rod_label_clip (Autodesk Fusion 360 design; units mm, degrees)
part number: 2026-09-05-07-00-16-324
Autodesk Fusion 360 part; units mm, degrees
sketch "Ring" plane through (0, 0, 0) normal (0, 1, 0) x (1, 0, 0)
  circle A0 centre (0, 0) radius 17.05
  circle A1 centre (0, 0) radius 19.45
extrude "Ring (1)" add sketch "Ring" along normal mid plane 9
sketch "Mouth" plane through (0, 0, 0) normal (0, 1, 0) x (1, 0, 0)
  line L0 (0, 0) -> (27.6739, -10.0725)
  line L1 (27.6739, -10.0725) -> (0, -29.45)
  line L2 (0, -29.45) -> (-27.6739, -10.0725)
  line L3 (-27.6739, -10.0725) -> (0, 0)
extrude "Mouth (1)" cut sketch "Mouth" along normal mid plane 19
sketch "Stem" plane through (0, 0, 0) normal (0, 1, 0) x (1, 0, 0)
  line L0 (12.2002, 12.6727) -> (20.8457, 22.976)
  line L1 (20.8457, 22.976) -> (19.0072, 24.5187)
  line L2 (19.0072, 24.5187) -> (10.3617, 14.2154)
  line L3 (10.3617, 14.2154) -> (12.2002, 12.6727)
extrude "Stem (1)" add sketch "Stem" along normal mid plane 9
sketch "Label face" plane through (0, 0, 0) normal (0, 1, 0) x (1, 0, 0)
  line L0 (20.8457, 22.976) -> (39.4865, 45.1913)
  line L1 (39.4865, 45.1913) -> (37.648, 46.734)
  line L2 (37.648, 46.734) -> (19.0072, 24.5187)
  line L3 (19.0072, 24.5187) -> (20.8457, 22.976)
extrude "Label face (1)" add sketch "Label face" along normal mid plane 58
equation "clipWidth = 9.0 mm" comment "drives the model; safe to edit live in Fusion"
equation "faceWidth = 58.0 mm" comment "drives the model; safe to edit live in Fusion"
equation "rodOuterDiameter = 33.4 mm" comment "reference only â edit scripts/build_rod_label_clip.py and rebuild"
equation "clipClearance = 0.7 mm" comment "reference only â edit scripts/build_rod_label_clip.py and rebuild"
equation "clipWall = 2.4 mm" comment "reference only â edit scripts/build_rod_label_clip.py and rebuild"
equation "mouthHalfAngleDeg = 70.0 mm" comment "reference only â edit scripts/build_rod_label_clip.py and rebuild"
equation "paddleAngleDeg = -50.0 mm" comment "reference only â edit scripts/build_rod_label_clip.py and rebuild"
equation "paddleThickness = 2.4 mm" comment "reference only â edit scripts/build_rod_label_clip.py and rebuild"
equation "stemEndRadius = 31.0 mm" comment "reference only â edit scripts/build_rod_label_clip.py and rebuild"
equation "faceEndRadius = 60.0 mm" comment "reference only â edit scripts/build_rod_label_clip.py and rebuild"
equation "d19 = clipWidth"
equation "d21 = clipWidth + 10 mm"
equation "d23 = clipWidth"
equation "d25 = faceWidth"
named bodies: "rod_label_clip"
